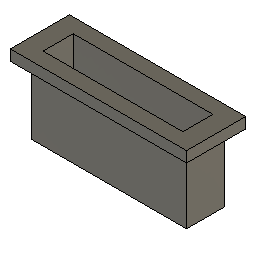
Amphenol G875H10620DEU compatible 3D printed connector for dupont 2.0 (Autodesk Fusion 360 design; units mm, degrees)
Autodesk Fusion 360 part; units mm, degrees
sketch "Sketch1" plane through (0, 0, 0) normal (0, 0, 1) x (1, 0, 0)
  line L0 (7.2, -1.75) -> (-7.2, -1.75)
  line L1 (-7.2, -1.75) -> (-7.2, 1.75)
  line L2 (-7.2, 1.75) -> (7.2, 1.75)
  line L3 (7.2, 1.75) -> (7.2, -1.75)
  line L4 (7.2, -1.75) -> (-7.2, 1.75) construction
  line L5 (-7.2, -1.75) -> (7.2, 1.75) construction
  line L6 (0.95, 2.75) -> (-0.95, 2.75)
  line L7 (-0.95, 2.75) -> (-0.95, 0.75)
  line L8 (-0.95, 0.75) -> (0.95, 0.75)
  line L9 (0.95, 0.75) -> (0.95, 2.75)
  line L10 (0.95, 2.75) -> (-0.95, 0.75) construction
  line L11 (-0.95, 2.75) -> (0.95, 0.75) construction
  line L12 (6.35, 1.25) -> (-6.35, 1.25)
  line L13 (-6.35, 1.25) -> (-6.35, -1.25)
  line L14 (-6.35, -1.25) -> (6.35, -1.25)
  line L15 (6.35, -1.25) -> (6.35, 1.25)
  line L16 (6.35, 1.25) -> (-6.35, -1.25) construction
  line L17 (-6.35, 1.25) -> (6.35, -1.25) construction
  line L18 (-6.5, -1.4) -> (6.5, -1.4)
  line L19 (6.5, -1.4) -> (6.5, 1.4)
  line L20 (6.5, 1.4) -> (-6.5, 1.4)
  line L21 (-6.5, 1.4) -> (-6.5, -1.4)
  point P0 (0, 1.75)
  dimension "d1" = 14.4
  dimension "d2" = 3.5
  dimension "d3" = 1.9
  dimension "d4" = 2
  dimension "d5" = 12.7
  dimension "d6" = 2.5
  dimension "d7" = 0.15
  constraint horizontal L0
  constraint perpendicular L0 L1
  constraint parallel L0 L2
  constraint parallel L1 L3
  constraint coincident L4 origin
  constraint coincident L5 origin
  constraint horizontal L6
  constraint perpendicular L6 L7
  constraint parallel L6 L8
  constraint parallel L7 L9
  constraint coincident L10 P0
  constraint coincident L11 P0
  constraint midpoint L2 P0
  constraint horizontal L12
  constraint perpendicular L12 L13
  constraint parallel L12 L14
  constraint parallel L13 L15
  constraint coincident L16 origin
  constraint coincident L17 origin
  measures "d1" distance of L1.end L2.end
  measures "d2" distance of L0.end L1.end
  measures "d3" distance of L7.end L8.end
  measures "d4" distance of L6.end L7.end
  measures "d5" distance of L13.end L14.end
  measures "d6" distance of L12.end L13.end
extrude "Extrude1" add sketch "Sketch1" along normal blind 6.3 contours L0 L1 L2 L3 L7 L9 L18 L19 L20 L21 | L2 L7 L9 L20 | L2 L6 L7 L9
extrude "Extrude2" cut 1 faces at (0.3167, 2.0833, 6.3) along direction (0, 0, -1) blind 1
sketch "Sketch2" plane through (0, 0, 5.3) normal (0, 0, 1) x (-1, 0, 0)
  line L0 (6.5, 1.4) -> (6.5, -1.4)
  line L1 (6.5, -1.4) -> (-6.5, -1.4)
  line L2 (-6.5, -1.4) -> (-6.5, 1.4)
  line L3 (-6.5, 1.4) -> (6.5, 1.4)
  line L4 (-0.95, -2.75) -> (0.95, -2.75)
  line L5 (0.95, -2.75) -> (0.95, -1.75)
  line L6 (0.95, -1.75) -> (7.2, -1.75)
  line L7 (7.2, -1.75) -> (7.2, 1.75)
  line L8 (7.2, 1.75) -> (-7.2, 1.75)
  line L9 (-7.2, 1.75) -> (-7.2, -1.75)
  line L10 (-7.2, -1.75) -> (-0.95, -1.75)
  line L11 (-0.95, -1.75) -> (-0.95, -2.75)
  line L12 (7.2, -2.75) -> (-7.2, -2.75)
  line L13 (-7.2, -2.75) -> (-7.2, 2.75)
  line L14 (-7.2, 2.75) -> (7.2, 2.75)
  line L15 (7.2, 2.75) -> (7.2, -2.75)
  line L16 (7.2, -2.75) -> (-7.2, 2.75) construction
  line L17 (-7.2, -2.75) -> (7.2, 2.75) construction
  line L18 (7.2, 2.75) -> (8.2, 2.75)
  line L19 (8.2, 2.75) -> (8.2, -2.75)
  line L20 (8.2, -2.75) -> (7.2, -2.75)
  line L21 (7.2, -2.75) -> (7.2, 2.75)
  line L22 (-7.2, 2.75) -> (-8.2, 2.75)
  line L23 (-8.2, 2.75) -> (-8.2, -2.75)
  line L24 (-8.2, -2.75) -> (-7.2, -2.75)
  line L25 (-7.2, -2.75) -> (-7.2, 2.75)
  dimension "d12" = 14.4
  dimension "d13" = 1
  dimension "d14" = 5.5
  dimension "d15" = 1
  constraint horizontal L12
  constraint perpendicular L12 L13
  constraint parallel L12 L14
  constraint parallel L13 L15
  constraint coincident L16 origin
  constraint coincident L17 origin
  constraint horizontal L18
  constraint vertical L19
  constraint horizontal L20
  constraint vertical L21
  constraint horizontal L22
  constraint vertical L23
  constraint horizontal L24
  constraint vertical L25
  measures "d12" distance of L13.end L14.end
  measures "d13" distance of L14.end L18.end
  measures "d14" distance of L14.end L12.start
  measures "d15" distance of L13.end L22.end
extrude "Extrude3" add sketch "Sketch2" along normal blind 2
extrude "Extrude4" cut 1 faces at (2.4, -2.4167, 5.3) along direction (0, 0, 1) blind 0.5
chamfer "Chamfer1" distance 0.5 angle 45 1 faces at (2.4, -2.4167, 5.8)
chamfer "Chamfer2" distance 0.25 angle 45 4 edges at (0, 1.4, 7.3) (6.5, 0, 7.3) (0, -1.4, 7.3) (-6.5, 0, 7.3)
sketch "Sketch3" plane through (0, 0, 0) normal (0, 0, -1) x (1, 0, 0)
  line L0 (-6.5, -1.4) -> (-6.5, 1.4)
  line L1 (-6.5, 1.4) -> (6.5, 1.4)
  line L2 (6.5, 1.4) -> (6.5, -1.4)
  line L3 (6.5, -1.4) -> (-6.5, -1.4)
  line L4 (-0.95, -2.75) -> (0.95, -2.75)
  line L5 (0.95, -2.75) -> (0.95, -1.75)
  line L6 (0.95, -1.75) -> (7.2, -1.75)
  line L7 (7.2, -1.75) -> (7.2, 1.75)
  line L8 (7.2, 1.75) -> (-7.2, 1.75)
  line L9 (-7.2, 1.75) -> (-7.2, -1.75)
  line L10 (-7.2, -1.75) -> (-0.95, -1.75)
  line L11 (-0.95, -1.75) -> (-0.95, -2.75)
  line L12 (-0.95, -2.75) -> (0.95, -2.75)
  line L13 (0.95, -2.75) -> (0.95, -1.75)
  line L14 (0.95, -1.75) -> (-0.95, -1.75)
  line L15 (-0.95, -1.75) -> (-0.95, -2.75)
  constraint horizontal L12
  constraint vertical L13
  constraint horizontal L14
  constraint vertical L15
  constraint coincident L5.end L6.start
  constraint coincident L4.start L11.end
extrude "Extrude5" cut sketch "Sketch3" against normal blind 0.5 contours L4 L5 L11 L12 L13 L14 L15
fillet "Fillet1" radius 0.55 2 edges at (0.95, 2.25, 0.5) (-0.95, 2.25, 0.5)
sketch "Sketch4" plane through (0, 0, 0) normal (0, 0, -1) x (1, 0, 0)
  line L0 (-7.2, -1.75) -> (7.2, -1.75)
  line L1 (7.2, -1.75) -> (7.2, 1.75)
  line L2 (7.2, 1.75) -> (-7.2, 1.75)
  line L3 (-7.2, 1.75) -> (-7.2, -1.75)
  line L4 (-6.5, -1.4) -> (-6.5, 1.4)
  line L5 (-6.5, 1.4) -> (6.5, 1.4)
  line L6 (6.5, 1.4) -> (6.5, -1.4)
  line L7 (6.5, -1.4) -> (-6.5, -1.4)
  line L8 (7.2, -1.75) -> (-7.2, -1.75)
  line L9 (-7.2, -1.75) -> (-7.2, 1.75)
  line L10 (-7.2, 1.75) -> (7.2, 1.75)
  line L11 (7.2, 1.75) -> (7.2, -1.75)
  line L12 (7.2, -1.75) -> (-7.2, 1.75) construction
  line L13 (-7.2, -1.75) -> (7.2, 1.75) construction
  line L14 (6.5, -1.4) -> (-6.5, -1.4)
  line L15 (-6.5, -1.4) -> (-6.5, 1.4)
  line L16 (-6.5, 1.4) -> (6.5, 1.4)
  line L17 (6.5, 1.4) -> (6.5, -1.4)
  line L18 (6.5, -1.4) -> (-6.5, 1.4) construction
  line L19 (-6.5, -1.4) -> (6.5, 1.4) construction
  line L20 (-5.8, 0.7) -> (5.8, 0.7)
  line L21 (5.8, 0.7) -> (5.8, -0.7)
  line L22 (5.8, -0.7) -> (-5.8, -0.7)
  line L23 (-5.8, -0.7) -> (-5.8, 0.7)
  dimension "d26" = 0.7
  constraint horizontal L8
  constraint perpendicular L8 L9
  constraint parallel L8 L10
  constraint parallel L9 L11
  constraint coincident L12 origin
  constraint coincident L13 origin
  constraint coincident L0.end L1.start
  constraint horizontal L14
  constraint perpendicular L14 L15
  constraint parallel L14 L16
  constraint parallel L15 L17
  constraint coincident L18 origin
  constraint coincident L19 origin
  constraint coincident L6.end L7.start
extrude "Extrude6" add sketch "Sketch4" against normal blind 0.7 contours L4 L5 L6 L7 L14 L15 L16 L17
chamfer "Chamfer3" distance 0.7 angle 45 4 edges at (0, 1.4, 0.7) (6.5, 0, 0.7) (0, -1.4, 0.7) (-6.5, 0, 0.7)
sketch "Sketch5" plane through (0, 0, 7.3) normal (0, 0, 1) x (-1, 0, 0)
  line L0 (8.2, 2.75) -> (-8.2, 2.75)
  line L1 (-8.2, 2.75) -> (-8.2, -2.75)
  line L2 (-8.2, -2.75) -> (8.2, -2.75)
  line L3 (8.2, -2.75) -> (8.2, 2.75)
  line L4 (-6.75, 1.65) -> (6.75, 1.65)
  line L5 (6.75, 1.65) -> (6.75, -1.65)
  line L6 (6.75, -1.65) -> (-6.75, -1.65)
  line L7 (-6.75, -1.65) -> (-6.75, 1.65)
  line L8 (-1.25, 2.75) -> (1.25, 2.75)
  line L9 (1.25, 2.75) -> (1.25, -2.75)
  line L10 (1.25, -2.75) -> (-1.25, -2.75)
  line L11 (-1.25, -2.75) -> (-1.25, 2.75)
  line L12 (-1.25, 2.75) -> (1.25, -2.75) construction
  line L13 (1.25, 2.75) -> (-1.25, -2.75) construction
  line L14 (-1.25, 2.75) -> (1.25, 2.75)
  line L15 (1.25, 2.75) -> (1.25, 1.65)
  line L16 (1.25, 1.65) -> (-1.25, 1.65)
  line L17 (-1.25, 1.65) -> (-1.25, 2.75)
  line L18 (-1.25, 1.65) -> (1.25, 1.65)
  line L19 (1.25, 1.65) -> (1.25, 0.65)
  line L20 (1.25, 0.65) -> (-1.25, 0.65)
  line L21 (-1.25, 0.65) -> (-1.25, 1.65)
  dimension "d30" = 2.5
  dimension "d31" = 1
  constraint horizontal L8
  constraint perpendicular L8 L9
  constraint parallel L8 L10
  constraint parallel L9 L11
  constraint coincident L12 origin
  constraint coincident L13 origin
  constraint horizontal L14
  constraint vertical L15
  constraint horizontal L16
  constraint vertical L17
  constraint coincident L9 L15.end
  constraint coincident L4 L15.end
  constraint horizontal L18
  constraint vertical L19
  constraint horizontal L20
  constraint vertical L21
  measures "d30" distance of L9.end L10.end
  measures "d31" distance of L16.end L20.end
extrude "Extrude7" add sketch "Sketch5" against normal blind 1 contours L4 L9 L11 L16 L18 L19 L20 L21
delete_face "DeleteFace1" 1 faces at (4.8333, -1.5667, 7.2167)
delete_face "DeleteFace2" 1 faces at (-4.8333, -1.5667, 7.2167)
delete_face "DeleteFace3" 1 faces at (-6.6667, 0.55, 7.2167)
delete_face "DeleteFace4" 1 faces at (2.25, 1.5667, 7.2167)
chamfer "Chamfer4" distance 0.4 angle 45 7 edges at (-6.5, 0, 7.3) (0.125, 1.4, 7.3) (-3.875, -1.4, 7.3) (-1.25, -1.025, 7.3) (0, -0.65, 7.3) (1.25, -1.025, 7.3) (4, -1.4, 7.3)
delete_face "DeleteFace5" 1 faces at (6.6667, 0.5167, 7.2167)
delete_face "DeleteFace6" 1 faces at (2.8667, -1.6667, 7.1667)
delete_face "DeleteFace7" 1 faces at (-3, -1.6667, 7.1667)
delete_face "DeleteFace8" 1 faces at (0.2833, -0.7833, 7.0333)
delete_face "DeleteFace9" 1 faces at (1.1167, -0.9, 7.0333)
delete_face "DeleteFace10" 1 faces at (-0.9833, -0.9, 7.1667)
delete_face "DeleteFace11" 1 faces at (-6.7667, 0.6, 7.1667)
delete_face "DeleteFace12" 1 faces at (-2.1667, 1.5333, 7.0333)
extrude "Extrude8" cut 1 faces at (-0.4167, -0.65, 6.9667) along direction (0, -1, 0) blind 0.25
chamfer "Chamfer5" distance 0.5 angle 45 1 edges at (0, -0.9, 7.3)
delete_face "DeleteFace13" 1 faces at (1.25, -1.2333, 6.8)
